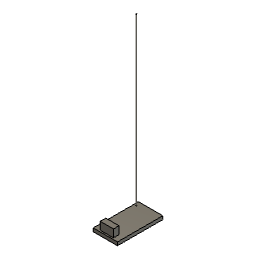
Lora Module (Autodesk Fusion 360 design; units mm, degrees)
Autodesk Fusion 360 part; units mm, degrees
sketch "Sketch1" plane through (0, 0, 0) normal (0, 1, 0) x (1, 0, 0)
  line L0 (0, 0) -> (22, 0)
  line L1 (22, 0) -> (22, -41)
  line L2 (22, -41) -> (0, -41)
  line L3 (0, -41) -> (0, 0)
  dimension "d1" = 22
  dimension "d2" = 41
  constraint horizontal L0
  constraint vertical L1
  constraint horizontal L2
  constraint vertical L3
  constraint coincident L0.start L3.end
  measures "d1" distance of L0.start L0.end
  measures "d2" distance of L0.start L2.end
extrude "Extrude1" add sketch "Sketch1" along normal blind 3
sketch "Sketch2" plane through (0, 3, 0) normal (0, 1, 0) x (-1, 0, 0)
  line L0 (0, 41) -> (-22, 41)
  line L1 (-22, 41) -> (-22, 0)
  line L2 (-22, 0) -> (0, 0)
  line L3 (0, 0) -> (0, 41)
  line L4 (-5, 34.6463) -> (-17, 34.6463)
  line L5 (-17, 34.6463) -> (-17, 39.6463)
  line L6 (-17, 39.6463) -> (-5, 39.6463)
  line L7 (-5, 39.6463) -> (-5, 34.6463)
  dimension "d5" = 12
  dimension "d6" = 5
  dimension "d7" = 5
  dimension "d8" = 5
  constraint horizontal L4
  constraint vertical L5
  constraint horizontal L6
  constraint vertical L7
  measures "d5" distance of L4.start L4.end
  measures "d6" distance of L4.start L6.end
  measures "d7" distance of L1 L5
  measures "d8" distance of L3 L7
extrude "Extrude2" add sketch "Sketch2" along normal blind 7 contours L4 L5 L6 L7
sketch "Sketch3" plane through (0, 3, 0) normal (0, 1, 0) x (-1, 0, 0)
  line L0 (-5, 39.6463) -> (-5, 34.6463)
  line L1 (-5, 34.6463) -> (-17, 34.6463)
  line L2 (-17, 34.6463) -> (-17, 39.6463)
  line L3 (-17, 39.6463) -> (-5, 39.6463)
  line L4 (0, 41) -> (-22, 41)
  line L5 (-22, 41) -> (-22, 0)
  line L6 (-22, 0) -> (0, 0)
  line L7 (0, 0) -> (0, 41)
  circle A0 centre (-2, 4) radius 0.5
  dimension "d11" = 1
  measures "d11" diameter of A0
extrude "Extrude3" add sketch "Sketch3" along normal blind 150 contours A0
